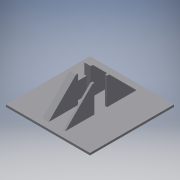
# Autodesk Inventor part: base
Saved by Autodesk Inventor 2018 (Build 220112000, 112)
## iProperties
Created: 2020-02-21
Part Number: base
Material: Generic
Document SubType Name: Modeling
Designer: bitbots
Density: 1 g/cm^3
Appearance: Default
Author: bitbots
Autodesk Inventor part; units mm, degrees
ref_plane "YZ Plane" through (0, 0, 0) normal (1, 0, 0) x (0, 1, 0)
ref_plane "XZ Plane" through (0, 0, 0) normal (0, 1, 0) x (-1, 0, 0)
ref_plane "XY Plane" through (0, 0, 0) normal (0, 0, 1) x (1, 0, 0)
sketch "Sketch1" plane through (0, 0, 0) normal (0, 0, 1) x (1, 0, 0)
  line L0 (-100, 100) -> (100, 100)
  line L1 (100, 100) -> (100, -100)
  line L2 (100, -100) -> (-100, -100)
  line L3 (-100, -100) -> (-100, 100)
  line L4 (-100, 100) -> (100, -100) construction
  line L5 (100, 100) -> (-100, -100) construction
  point P0 (0, 0)
  dimension "d0" = 200
  dimension "d1" = 200
  constraints: 12 end point, 2 midpoint, 2 parallel, 1 horizontal, 1 perpendicular
  measures "d0" distance of L1.end L2.end
  measures "d1" distance of L0.end L1.end
extrude "Extrusion1" add sketch "Sketch1" along normal blind 5
ref_plane "Work Plane1" through (-17.3121, -15, 70.1) normal (0, 0, 1) x (1, 0, 0)
sketch "Sketch3" plane through (0, 0, 5) normal (0, 0, 1) x (1, 0, 0)
  line L0 (-13.3095, -15) -> (-13.3095, -20.1)
  line L1 (-13.3095, -14.5) -> (-18.3095, -14.5)
  line L2 (20.6905, -15) -> (20.6905, -20.1)
  line L3 (25.6905, -14.5) -> (20.6905, -14.5)
  line L4 (-13.3095, 20.1) -> (-13.3095, 15)
  line L5 (-18.3095, 14.5) -> (-13.3095, 14.5)
  line L6 (20.6905, 20.1) -> (20.6905, 15)
  line L7 (25.6905, 14.5) -> (20.6905, 14.5)
  line L8 (20.6905, -15) -> (25.6905, -15)
  line L9 (25.6905, -15) -> (25.6905, -20)
  line L10 (25.6905, -20) -> (20.6905, -20)
  line L11 (20.6905, -20) -> (20.6905, -15)
  line L12 (-13.3095, -20.1) -> (-28.3095, -20.1)
  line L13 (-28.3095, -20.1) -> (-28.3095, -15.1)
  line L14 (-28.3095, -15.1) -> (-13.3095, -15.1)
  line L15 (-13.3095, -15.1) -> (-13.3095, -20.1)
  line L16 (-13.3095, 20.1) -> (-28.3095, 20.1)
  line L17 (-28.3095, 20.1) -> (-28.3095, 15.1)
  line L18 (-28.3095, 15.1) -> (-13.3095, 15.1)
  line L19 (-13.3095, 15.1) -> (-13.3095, 20.1)
  line L20 (20.6905, 20.1) -> (25.6905, 20.1)
  line L21 (25.6905, 20.1) -> (25.6905, 15.1)
  line L22 (25.6905, 15.1) -> (20.6905, 15.1)
  line L23 (20.6905, 15.1) -> (20.6905, 20.1)
  point P0 (0, 0)
extrude "Extrusion2" add sketch "Sketch3" along normal up to surface (65.1 mm away)
chamfer "Chamfer1" distance 65.1 angle 45 5 edges at (-20.8095, 20.1, 5) (23.1905, 20.1, 5) (-28.3095, -20.1, 37.55) (-20.8095, -20.1, 5) (23.1905, -20, 5)
sketch "Sketch4" plane through (-28.3095, 15.1, 5) normal (-1, 0, 0) x (0, 0, 1)
  line L0 (0, 0) -> (65.1, 0) projected
  line L1 (65.1, 0) -> (40.1, 0)
  line L2 (65.1, 0) -> (90.1, 0) construction
  line L3 (0, -30.2) -> (65.1, -30.2) projected
  line L4 (40.1, 0) -> (0, 0)
  line L5 (0, 0) -> (0, -30.2)
  line L6 (0, -30.2) -> (40.1, -30.2)
  line L7 (40.1, -30.2) -> (40.1, 0)
  point P0 (-5, -15.1)
  dimension "d17" = 25
  dimension "d18" = 180
  constraints: 12 end point, 2 collinear, 2 horizontal, 2 parallel, 1 perpendicular
  measures "d17" distance of L0.end L1.end
  measures "d18" angle of L1 L2
extrude "Extrusion3" add sketch "Sketch4" against normal blind 5
body "Solid1"
